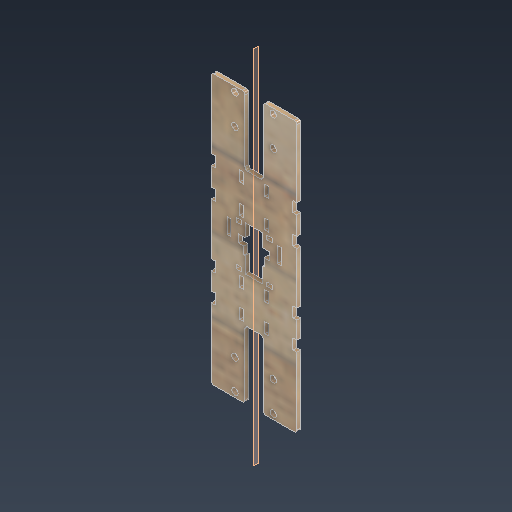
# Autodesk Inventor part: main_frame
Saved by Autodesk Inventor 2025.3 (Build 293356000, 356)
## iProperties
Created: 2025-09-03
Part Number: main_frame
Material: 木材 (楓木)
Document SubType Name: Modeling
Designer: 陳泓任
Density: 0.67 g/cm^3
Appearance: 天然楓木 - 深色亮面處理
Author: 陳泓任
Autodesk Inventor part; units mm, degrees
ref_plane "XZ Plane" through (0, 0, 0) normal (0, 1, 0) x (-1, 0, 0)
ref_plane "XY Plane" through (0, 0, 0) normal (0, 0, 1) x (1, 0, 0)
sketch "草圖1" plane through (0, 0, 0) normal (0, 0, 1) x (1, 0, 0)
  line L0 (-33, -104) -> (33, 104) construction
  line L1 (33, -104) -> (-33, 104) construction
  line L2 (0, 128.5379) -> (0, -160.5456) construction
  circle A0 centre (-14.75, 100) radius 2.5
  circle A1 centre (14.75, 100) radius 2.5
  circle A2 centre (14.75, 77) radius 2.5
  circle A3 centre (-14.75, 77) radius 2.5
  line L3 (-33, 49.8787) -> (-30, 49.8787)
  line L4 (-30, 49.8787) -> (-30, 41.8787)
  line L5 (-30, 41.8787) -> (-33, 41.8787)
  line L6 (-33, 102) -> (-33, 49.8787)
  line L7 (-11.2, 49.8787) -> (-8.2, 49.8787)
  line L8 (-8.2, 49.8787) -> (-8.2, 41.8787)
  line L9 (-8.2, 41.8787) -> (-11.2, 41.8787)
  line L10 (-11.2, 41.8787) -> (-11.2, 49.8787)
  line L11 (33, 49.8787) -> (30, 49.8787)
  line L12 (30, 49.8787) -> (30, 41.8787)
  line L13 (30, 41.8787) -> (33, 41.8787)
  line L14 (11.2, 49.8787) -> (8.2, 49.8787)
  line L15 (8.2, 49.8787) -> (8.2, 41.8787)
  line L16 (8.2, 41.8787) -> (11.2, 41.8787)
  line L17 (11.2, 41.8787) -> (11.2, 49.8787)
  line L18 (33, 49.8787) -> (33, 102)
  line L19 (-33, 41.8787) -> (-33, 27.4291)
  line L20 (33, 27.4291) -> (33, 41.8787)
  line L21 (-5, 52) -> (5, 52)
  line L22 (7, 54) -> (7, 102)
  line L23 (-7, 102) -> (-7, 54)
  line L24 (-7, 52) -> (7, 104) construction
  line L25 (7, 52) -> (-7, 104) construction
  line L26 (31, 104) -> (9, 104)
  line L27 (-9, 104) -> (-31, 104)
  arc A4 (-7, 102) -> (-9, 104) centre (-9, 102) ccw
  arc A5 (9, 104) -> (7, 102) centre (9, 102) ccw
  arc A6 (-7, 54) -> (-5, 52) centre (-5, 54) ccw
  arc A7 (5, 52) -> (7, 54) centre (5, 54) ccw
  arc A8 (-31, 104) -> (-33, 102) centre (-31, 102) ccw
  arc A9 (33, 102) -> (31, 104) centre (31, 102) ccw
  line L28 (-82.8249, 0) -> (86.4934, 0) construction
  circle A10 centre (-14.75, -100) radius 2.5
  circle A11 centre (14.75, -100) radius 2.5
  circle A12 centre (14.75, -77) radius 2.5
  circle A13 centre (-14.75, -77) radius 2.5
  line L29 (-33, -49.8787) -> (-30, -49.8787)
  line L30 (-30, -49.8787) -> (-30, -41.8787)
  line L31 (-30, -41.8787) -> (-33, -41.8787)
  line L32 (-33, -102) -> (-33, -49.8787)
  line L33 (-11.2, -49.8787) -> (-8.2, -49.8787)
  line L34 (-8.2, -49.8787) -> (-8.2, -41.8787)
  line L35 (-8.2, -41.8787) -> (-11.2, -41.8787)
  line L36 (-11.2, -41.8787) -> (-11.2, -49.8787)
  line L37 (33, -49.8787) -> (30, -49.8787)
  line L38 (30, -49.8787) -> (30, -41.8787)
  line L39 (30, -41.8787) -> (33, -41.8787)
  line L40 (8.2, -41.8787) -> (11.2, -41.8787)
  line L41 (11.2, -41.8787) -> (11.2, -49.8787)
  line L42 (8.2, -49.8787) -> (8.2, -41.8787)
  line L43 (11.2, -49.8787) -> (8.2, -49.8787)
  line L44 (33, -49.8787) -> (33, -102)
  line L45 (8.2, -28.45) -> (8.2, -20.45)
  line L46 (8.2, -20.45) -> (11.2, -20.45)
  line L47 (11.2, -28.45) -> (8.2, -28.45)
  line L48 (11.2, -20.45) -> (11.2, -28.45)
  line L49 (30, -28.45) -> (30, -20.45)
  line L50 (30, -20.45) -> (33, -20.45)
  line L51 (33, -28.45) -> (30, -28.45)
  line L52 (-8.2, -28.45) -> (-8.2, -20.45)
  line L53 (-8.2, -20.45) -> (-11.2, -20.45)
  line L54 (-11.2, -28.45) -> (-8.2, -28.45)
  line L55 (-11.2, -20.45) -> (-11.2, -28.45)
  line L56 (-30, -28.45) -> (-30, -20.45)
  line L57 (-33, -28.45) -> (-30, -28.45)
  line L58 (-30, -20.45) -> (-33, -20.45)
  line L59 (-33, -41.8787) -> (-33, -28.45)
  line L60 (33, -28.45) -> (33, -41.8787)
  line L61 (-5, -52) -> (5, -52)
  line L62 (7, -54) -> (7, -102)
  line L63 (-7, -102) -> (-7, -54)
  line L64 (-7, -52) -> (7, -104) construction
  line L65 (7, -52) -> (-7, -104) construction
  line L66 (31, -104) -> (9, -104)
  line L67 (-9, -104) -> (-31, -104)
  arc A14 (-9, -104) -> (-7, -102) centre (-9, -102) ccw
  arc A15 (7, -102) -> (9, -104) centre (9, -102) ccw
  arc A16 (-5, -52) -> (-7, -54) centre (-5, -54) ccw
  arc A17 (7, -54) -> (5, -52) centre (5, -54) ccw
  arc A18 (-33, -102) -> (-31, -104) centre (-31, -102) ccw
  arc A19 (31, -104) -> (33, -102) centre (31, -102) ccw
  line L68 (-31, -104) -> (-9, -104)
  line L69 (9, -104) -> (31, -104)
  line L70 (-6.85, -17.45) -> (6.85, -17.45)
  line L71 (6.85, 16.75) -> (-6.85, 16.75)
  line L72 (12.065, 0.7) -> (12.065, 6.7)
  line L73 (-12.065, 6.7) -> (-12.065, 0.7)
  line L74 (-12.065, 0.7) -> (12.065, 6.7) construction
  line L75 (12.065, 0.7) -> (-12.065, 6.7) construction
  line L76 (-6.85, 16.75) -> (-6.85, 6.7)
  line L77 (6.85, 6.7) -> (6.85, 16.75)
  line L78 (12.065, 6.7) -> (6.85, 6.7)
  line L79 (7.85, 0.7) -> (12.065, 0.7)
  line L80 (-12.065, 0.7) -> (-7.85, 0.7)
  line L81 (-6.85, 6.7) -> (-12.065, 6.7)
  line L82 (-33, -28.45) -> (-33, -41.8787)
  line L83 (-33, -49.8787) -> (-33, -102)
  line L84 (33, -102) -> (33, -49.8787)
  line L85 (33, -41.8787) -> (33, -28.45)
  line L86 (-11.2, -41.8787) -> (-8.2, -49.8787) construction
  line L87 (-8.2, -41.8787) -> (-11.2, -49.8787) construction
  line L88 (-13.3213, -39.7574) -> (-6.0787, -39.7574) construction
  line L89 (-6.0787, -39.7574) -> (-6.0787, -52) construction
  line L90 (-6.0787, -52) -> (-13.3213, -52) construction
  line L91 (-13.3213, -52) -> (-13.3213, -39.7574) construction
  line L92 (-8.2, -41.8787) -> (-6.0787, -39.7574) construction
  circle A20 centre (-6.85, 16.75) radius 3 construction
  line L93 (-11.2, 27.4291) -> (-8.2, 27.4291)
  line L94 (-8.2, 27.4291) -> (-8.2, 19.4291)
  line L95 (-8.2, 19.4291) -> (-11.2, 19.4291)
  line L96 (-11.2, 19.4291) -> (-11.2, 27.4291)
  line L97 (-33, 27.4291) -> (-30, 27.4291)
  line L98 (-30, 27.4291) -> (-30, 19.4291)
  line L99 (-30, 19.4291) -> (-33, 19.4291)
  line L100 (11.2, 27.4291) -> (8.2, 27.4291)
  line L101 (8.2, 27.4291) -> (8.2, 19.4291)
  line L102 (8.2, 19.4291) -> (11.2, 19.4291)
  line L103 (11.2, 19.4291) -> (11.2, 27.4291)
  line L104 (33, 27.4291) -> (30, 27.4291)
  line L105 (30, 27.4291) -> (30, 19.4291)
  line L106 (30, 19.4291) -> (33, 19.4291)
  line L107 (-33, 19.4291) -> (-33, -20.45)
  line L108 (33, 19.4291) -> (33, -20.45)
  line L109 (-9.85, -17.45) -> (-14.15, -17.45) construction
  line L110 (-14.15, -17.45) -> (-14.15, -14.45) construction
  line L111 (-14.15, -14.45) -> (-9.85, -14.45) construction
  line L112 (-9.85, -14.45) -> (-9.85, -17.45) construction
  line L113 (-17.15, -20.45) -> (-6.85, -20.45) construction
  line L114 (-6.85, -20.45) -> (-6.85, -11.45) construction
  line L115 (-6.85, -11.45) -> (-17.15, -11.45) construction
  line L116 (-17.15, -11.45) -> (-17.15, -20.45) construction
  line L117 (-7.85, 0.7) -> (-7.85, -5.3)
  line L118 (-7.85, -5.3) -> (-6.85, -5.3)
  line L119 (-6.85, -5.3) -> (-6.85, -17.45)
  line L120 (7.85, 0.7) -> (7.85, -5.3)
  line L121 (7.85, -5.3) -> (6.85, -5.3)
  line L122 (6.85, -17.45) -> (6.85, -5.3)
  point P0 (0, 0)
  point P1 (0, 86.5078)
  point P2 (0, 78)
  point P3 (0, -86.5078)
  point P4 (0, -78)
  point P5 (0, 3.7)
  point P6 (12.065, 3.7)
  dimension "d56" = 6
  dimension "d0" = 66
  dimension "d1" = 208
  dimension "d6" = 5
  dimension "d8" = 29.5
  dimension "d9" = 23
  dimension "d10" = 3
  dimension "d11" = 8
  dimension "d13" = 3
  dimension "d14" = 18.8
  dimension "d22" = 14
  dimension "d23" = 4
  dimension "d24" = 2
  dimension "d25" = 2
  dimension "d26" = 34.2
  dimension "d27" = 13.7
  dimension "d28" = 6
  dimension "d30" = 24.13
  dimension "d31" = 10.05
  dimension "d53" = 3
  dimension "d54" = 52
  dimension "d57" = 3
  dimension "d58" = 3
  dimension "d71" = 4.3
  dimension "d73" = 3
  dimension "d74" = 3
  dimension "d97" = 6
  dimension "d98" = 1
  dimension "d101" = 0.7
  constraints: 246 end point, 63 symmetric about line, 42 parallel, 29 point on line, 24 perpendicular, 24 point on circle, 20 centre point, 16 collinear, 15 horizontal, 12 tangent, 11 equal length, 7 equal radius, 7 midpoint, 4 vertical, 1 coincident, 1 vertical alignment, 23 other
  measures "d0" distance of L0.end L1.end
  measures "d1" distance of L1.start L0.end
  measures "d6" diameter of A0
  measures "d8" distance of A2.centre A3.centre
  measures "d9" distance of A1.centre A2.centre
  measures "d10" distance of L4.end L5.end
  measures "d11" distance of L3.end L4.end
  measures "d13" distance of L7.start L7.end
  measures "d14" distance between parallel lines of L4 L10
  measures "d22" distance of L24.start L25.start
  measures "d23" distance from line of A0.centre L27
  measures "d24" radius of A4
  measures "d25" radius of A8
  measures "d26" distance of L70.end L71.start
  measures "d27" distance of L71.start L71.end
  measures "d28" distance of L72.start L72.end
  measures "d30" distance from line of point (12.065, 3.7) L73
  measures "d31" distance between parallel lines of L81 L71
  measures "d53" distance of L35.start L88.end
  measures "d54" distance between parallel lines of L27 L21
  measures "d57" distance of L93.start L93.end
  measures "d58" distance of L19.end L97.end
  measures "d71" distance of L110.end L111.end
  measures "d73" distance of L109.end L110.end
  measures "d74" distance between parallel lines of L109 L113
  measures "d97" distance of L80.end L117.end
  measures "d98" distance of L117.end L118.end
  measures "d101" distance between parallel lines of L28 L80
extrude "擠出1" add sketch "草圖1" along normal blind 3
sketch "草圖3" plane through (0, 0, 3) normal (0, 0, 1) x (1, 0, 0)
  line L0 (-88.1264, 0) -> (75.7938, 0)
  line L1 (0, 123.8394) -> (0, -129.4918)
  point P0 (0, 0)
  constraints: 4 end point, 2 point on line, 1 horizontal, 1 perpendicular
sketch "草圖5" plane through (0, 0, 3) normal (0, 0, 1) x (1, 0, 0)
  line L0 (-9.85, -17.45) -> (-13.85, -17.45)
  line L1 (-13.85, -17.45) -> (-13.85, -14.45)
  line L2 (-13.85, -14.45) -> (-9.85, -14.45)
  line L3 (-9.85, -14.45) -> (-9.85, -17.45)
  line L4 (6.85, -17.45) -> (-6.85, -17.45) projected
  line L5 (-9.85, 13.75) -> (-13.85, 13.75)
  line L6 (-13.85, 13.75) -> (-13.85, 16.75)
  line L7 (-13.85, 16.75) -> (-9.85, 16.75)
  line L8 (-9.85, 16.75) -> (-9.85, 13.75)
  line L9 (-6.85, 16.75) -> (6.85, 16.75) projected
  line L10 (0, 31.1544) -> (0, -25.4134)
  line L11 (9.85, -17.45) -> (13.85, -17.45)
  line L12 (13.85, -17.45) -> (13.85, -14.45)
  line L13 (13.85, -14.45) -> (9.85, -14.45)
  line L14 (9.85, -14.45) -> (9.85, -17.45)
  line L15 (13.85, 16.75) -> (9.85, 16.75)
  line L16 (13.85, 13.75) -> (13.85, 16.75)
  line L17 (9.85, 13.75) -> (13.85, 13.75)
  line L18 (9.85, 16.75) -> (9.85, 13.75)
  line L19 (-17.85, 1.825) -> (-20.85, 1.825)
  line L20 (-20.85, 1.825) -> (-20.85, 13.825)
  line L21 (-20.85, 13.825) -> (-17.85, 13.825)
  line L22 (-17.85, 13.825) -> (-17.85, 1.825)
  line L23 (17.85, 1.825) -> (20.85, 1.825)
  line L24 (20.85, 1.825) -> (20.85, 13.825)
  line L25 (20.85, 13.825) -> (17.85, 13.825)
  line L26 (17.85, 13.825) -> (17.85, 1.825)
  line L27 (-6.85, -17.45) -> (-6.85, 16.75) construction
  point P0 (0, 0)
  dimension "d60" = 4
  dimension "d62" = 3
  dimension "d64" = 3
  dimension "d66" = 3
  dimension "d67" = 12
  dimension "d96" = 3
  dimension "d100" = 11
  dimension "d102" = 0.075
  constraints: 52 end point, 12 symmetric about line, 6 parallel, 4 collinear, 3 horizontal, 3 perpendicular, 1 point on line, 1 vertical
  measures "d60" distance of L0.start L0.end
  measures "d62" distance of L0.end L1.end
  measures "d64" distance of L6.start L7.start
  measures "d66" distance of L20.end L21.end
  measures "d67" distance of L21.end L19.start
  measures "d96" distance between parallel lines of L27 L3
  measures "d100" distance between parallel lines of L27 L22
  measures "d102" distance between parallel lines of L5 L21
extrude "擠出4" cut sketch "草圖5" against normal up to next
